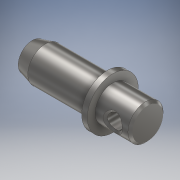
# Autodesk Inventor part: Pin_RBF
Saved by Autodesk Inventor 2017 (Build 210142000, 142)
## iProperties
Created: 2018-05-13
Part Number: Pin_RBF
Material: Stainless Steel
Document SubType Name: Modeling
Designer: Bradley
Stock Number: 98470A002
Density: 8 g/cm^3
Appearance: Semi-Polished
Author: Bradley
Autodesk Inventor part; units mm, degrees
ref_plane "YZ Plane" through (0, 0, 0) normal (1, 0, 0) x (0, 1, 0)
ref_plane "XZ Plane" through (0, 0, 0) normal (0, 1, 0) x (-1, 0, 0)
ref_plane "XY Plane" through (0, 0, 0) normal (0, 0, 1) x (1, 0, 0)
sketch "Sketch1" plane through (0, 0, 0) normal (0, 0, 1) x (1, 0, 0)
  line L0 (-7.83, 0) -> (7.83, 0)
  line L1 (7.83, 0) -> (7.83, 2.3813)
  line L2 (7.83, 2.3813) -> (3.092, 2.3813)
  line L3 (3.092, 2.3813) -> (3.092, 3.4544)
  line L4 (3.092, 3.4544) -> (2.33, 3.4544)
  line L5 (2.33, 3.4544) -> (2.33, 2.3813)
  line L6 (2.33, 2.3813) -> (-6.052, 2.3812)
  line L7 (-6.052, 2.3812) -> (-7.83, 1.905)
  line L8 (-7.83, 1.905) -> (-7.83, 0)
  point P0 (0, 0)
  point P1 (0, 0)
  dimension "d0" = 4.7625
  dimension "d1" = 10.16
  dimension "d2" = 6.9088
  dimension "d3" = 1.778
  dimension "d4" = 3.81
  dimension "d5" = 0.762
  dimension "d6" = 5.5
  dimension "d7" = 4.738
  constraints: 18 end point, 5 perpendicular, 2 point on line, 1 coincident, 1 horizontal, 1 midpoint, 1 parallel
  measures "d0" diameter of L6 L0
  measures "d1" distance between parallel lines of L8 L5
  measures "d2" diameter of L4 L0
  measures "d3" horizontal distance of L6.end L7.end
  measures "d4" diameter of L7.end L0
  measures "d5" distance of L3.end L4.end
  measures "d6" distance between parallel lines of L1 L5
  measures "d7" distance of L1.end L2.end
revolve "Revolution1" add sketch "Sketch1" angle 360 about axis through (-7.83, 0, 0) along (1, 0, 0)
sketch "Sketch2" plane through (0, 0, 0) normal (0, 1, 0) x (-1, 0, 0)
  line L0 (-3.092, 2.3812) -> (-3.092, -2.3812) projected
  line L1 (-3.092, 0) -> (-7.83, 0) construction
  circle A0 centre (-5.461, 0) radius 1
  line L2 (-7.83, 2.3812) -> (-7.83, -2.3812) projected
  point P0 (0, 0)
  point P1 (-7.33, 2.3812)
  point P2 (-7.33, -2.3812)
  dimension "d12" = 2
  constraints: 3 midpoint, 2 end point, 1 centre point
  measures "d12" diameter of A0
extrude "Extrusion1" cut sketch "Sketch2" along normal through all both and the other way through all
chamfer "Chamfer2" distance 0.3 angle 45 4 edges at (7.83, -2.3812, 0) (5.4611, 2.1611, 1) (5.4609, 2.1611, -1) (6.461, -2.3812, -0.003)
sketch "Sketch3" plane through (0, 0, 0) normal (0, 0, 1) x (1, 0, 0)
  line L0 (-6.052, 2.3812) -> (2.33, 2.3812) projected
  line L1 (-7.83, -1.905) -> (-7.83, 1.905) projected
  arc A0 (-2.7246, 2.1654) -> (-3.9946, 2.1654) centre (-3.3596, 2.1654) ccw
  line L2 (-3.9946, 2.1654) -> (-2.7246, 2.1654)
  line L3 (-6.052, -2.3812) -> (2.33, -2.3812) projected
  line L4 (2.33, -3.4544) -> (2.33, 3.4544) projected
  point P0 (0, 0)
  point P1 (-3.3596, 2.8004)
  point P2 (-2.7624, 2.3812)
  dimension "d18" = 4.4704
  dimension "d20" = 5.1816
  dimension "d21" = 1.27
  dimension "d22" = 5.0924
  constraints: 4 point on circle, 2 end point, 1 centre point, 1 coincident, 1 horizontal, 1 midpoint, 1 point on line
  measures "d18" distance from line of L1 A0.centre
  measures "d20" distance from line of L3 point (-3.36, 2.8)
  measures "d21" distance of L2.start L2.end
  measures "d22" distance from line of L4 point (-2.762, 2.381)
revolve "Revolution2" add sketch "Sketch3" angle 360 about axis through (-3.9946, 2.1654, 0) along (1, 0, 0)
body "Solid1"
